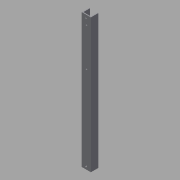
# Autodesk Inventor part: 18in C-Channel Front
Saved by Autodesk Inventor 2013 (Build 170138000, 138)
## iProperties
Created: 2013-01-08
Part Number: 18in C-Channel Front
Material: Aluminum 6061
Document SubType Name: Modeling
Designer: Naphat
Density: 1 g/cm^3
Author: Naphat
Autodesk Inventor part; units mm, degrees
ref_plane "YZ Plane" through (0, 0, 0) normal (1, 0, 0) x (0, 1, 0)
ref_plane "XZ Plane" through (0, 0, 0) normal (0, 1, 0) x (-1, 0, 0)
ref_plane "XY Plane" through (0, 0, 0) normal (0, 0, 1) x (1, 0, 0)
sketch "Sketch1" plane through (0, 0, 0) normal (0, 0, 1) x (1, 0, 0)
  line L0 (-15.7, 12.7) -> (-12.7, 12.7)
  line L1 (-12.7, 12.7) -> (-12.7, -9.7)
  line L2 (-12.7, -9.7) -> (12.7, -9.7)
  line L3 (12.7, -9.7) -> (12.7, 12.7)
  line L4 (12.7, 12.7) -> (15.7, 12.7)
  line L5 (15.7, 12.7) -> (15.7, -12.7)
  line L6 (15.7, -12.7) -> (-15.7, -12.7)
  line L7 (-15.7, -12.7) -> (-15.7, 12.7)
  point P0 (0, 0)
  dimension "d0" = 3
  dimension "d2" = 3
  dimension "d3" = 25.4
  dimension "d4" = 31.4
  dimension "d5" = 15.7
  dimension "d7" = 12.7
  dimension "d8" = 3
  constraints: 16 end point, 5 parallel, 1 collinear, 1 horizontal, 1 perpendicular
  measures "d0" distance of L0.start L0.end
  measures "d2" distance of L3.end L4.end
  measures "d3" distance of L6.end L0.start
  measures "d4" distance of L5.end L6.end
  measures "d5" distance from line of point (0, 0) L7
  measures "d7" distance from line of L6 point (0, 0)
  measures "d8" distance between parallel lines of L6 L2
extrude "Extrusion1" add sketch "Sketch1" against normal blind 457.2
sketch "Sketch7" plane through (-15.7, -12.7, 0) normal (0, -1, 0) x (1, 0, 0)
  circle A0 centre (13.8784, -447.9) radius 3.175
  point P0 (15.7, 0)
  dimension "d25" = 6.35
  constraints: 1 centre point
  measures "d25" diameter of A0
extrude "Extrusion5" cut sketch "Sketch7" against normal blind 10
sketch "Sketch8" plane through (-15.7, -12.7, 0) normal (0, -1, 0) x (1, 0, 0)
  line L0 (0, -184) -> (31.4, -184) construction
  line L1 (31.4, -134) -> (0, -134) construction
  line L2 (31.4, -134) -> (31.4, -184) construction
  line L3 (15.7, -134) -> (15.7, -159) construction
  line L4 (15.7, -159) -> (31.4, -159) construction
  circle A0 centre (15.7, -159) radius 3.175
  point P0 (15.7, 0)
  dimension "d29" = 6.35
  constraints: 10 end point, 2 midpoint, 1 centre point, 1 coincident, 1 parallel
  measures "d29" diameter of A0
extrude "Extrusion6" cut sketch "Sketch8" against normal blind 10
sketch "Sketch9" plane through (-15.7, -12.7, 0) normal (0, -1, 0) x (1, 0, 0)
  circle A0 centre (13.8784, -9.3) radius 3.175
  circle A1 centre (15.7, -29) radius 3.175
  point P0 (15.7, 0)
  constraints: 2 centre point
extrude "Extrusion7" cut sketch "Sketch9" against normal blind 10
equation "\"d2\" = d0"
equation "\"d5\" = 0.5 * d4"
equation "\"d7\" = 0.5 * d3"
equation "\"d8\" = d0"
body "Solid1"
